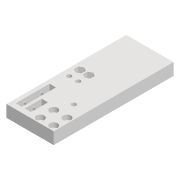
# Autodesk Inventor part: Fixed top coupler
Saved by Autodesk Inventor 2020 (Build 240168000, 168)
## iProperties
Created: 2019-10-02
Part Number: Fixed top coupler
Material: Generic
Document SubType Name: Modeling
Designer: ball
Density: 1 g/cm^3
Appearance: Default
Author: ball
Autodesk Inventor part; units mm, degrees
ref_plane "YZ Plane" through (0, 0, 0) normal (1, 0, 0) x (0, 1, 0)
ref_plane "XZ Plane" through (0, 0, 0) normal (0, 1, 0) x (-1, 0, 0)
ref_plane "XY Plane" through (0, 0, 0) normal (0, 0, 1) x (1, 0, 0)
sketch "Sketch1" plane through (0, 0, 0) normal (0, 1, 0) x (-1, 0, 0)
  line L0 (0, 0) -> (35.5, 0)
  line L1 (35.5, 0) -> (35.5, -90)
  line L2 (35.5, -90) -> (0, -90)
  line L3 (0, -90) -> (0, 0)
  dimension "d0" = 35.5
  dimension "d1" = 90
  constraints: 8 end point, 2 parallel, 1 horizontal, 1 perpendicular
  measures "d0" distance of L1.end L2.end
  measures "d1" distance of L0.end L1.end
extrude "Extrusion1" add sketch "Sketch1" along normal blind 9
sketch "Sketch3" plane through (0, 0, 0) normal (0, -1, 0) x (1, 0, 0)
  circle A0 centre (-10, -25) radius 3.25 construction
  line L0 (0, 0) -> (-35.5, 0) projected
  line L1 (-35.5, 0) -> (-35.5, -90) projected
  line L2 (-11.6286, -27.8125) -> (-13.25, -24.9958)
  line L3 (-13.25, -24.9958) -> (-11.6214, -22.1833)
  line L4 (-11.6214, -22.1833) -> (-8.3714, -22.1875)
  line L5 (-8.3714, -22.1875) -> (-6.75, -25.0042)
  line L6 (-6.75, -25.0042) -> (-8.3786, -27.8167)
  line L7 (-8.3786, -27.8167) -> (-11.6286, -27.8125)
  line L8 (0, -90) -> (0, 0) projected
  dimension "d15" = 6.5
  dimension "d16" = 25
  dimension "d26" = 10
  constraints: 12 end point, 1 coincident, 16 other
  measures "d16" distance from line of L0 point (-10, -25)
  measures "d26" distance from line of L8 point (-10, -25)
extrude "Extrusion3" cut sketch "Sketch3" against normal blind 5
sketch "Sketch5" plane through (0, 9, 0) normal (0, 1, 0) x (1, 0, 0)
  line L0 (0, 0) -> (0, 90) projected
  line L1 (-35.5, 0) -> (0, 0) projected
  circle A0 centre (-10, 25) radius 1.7
  dimension "d36" = 3.4
  dimension "d37" = 25
  constraints: 1 centre point
  measures "d36" diameter of A0
  measures "d37" distance from line of L1 A0.centre
extrude "Extrusion4" cut sketch "Sketch5" against normal through all
sketch "Sketch6" plane through (0, 9, 0) normal (0, 1, 0) x (1, 0, 0)
  line L0 (-32.5, 4) -> (-27.7502, 4)
  line L1 (-27.7502, 4) -> (-27.7502, 29.4)
  line L2 (-27.7502, 29.4) -> (-32.5, 29.4)
  line L3 (-32.5, 29.4) -> (-32.5, 4)
  line L4 (-35.5, 0) -> (0, 0) projected
  line L5 (-35.5, 90) -> (-35.5, 0) projected
  line L6 (-25.7502, 4) -> (-21.0002, 4)
  line L7 (-21.0002, 4) -> (-21.0002, 16.7)
  line L8 (-21.0002, 16.7) -> (-25.7502, 16.7)
  line L9 (-25.7502, 16.7) -> (-25.7502, 4)
  line L10 (0, 0) -> (0, 90) construction
  line L11 (-35.5, 90) -> (0, 90) projected
  line L12 (0, 0) -> (-20, 0) construction
  line L13 (-20, 0) -> (-20, 90) construction
  line L14 (-20, 90) -> (0, 90) construction
  line L15 (0, 90) -> (0, 0)
  circle A0 centre (-23.3752, 41.7) radius 1.7
  circle A1 centre (-30.125, 41.7) radius 1.7
  circle A2 centre (-30.125, 49.7) radius 1.7
  circle A3 centre (-23.3752, 49.7) radius 1.7
  dimension "d43" = 4.7498
  dimension "d44" = 25.4
  dimension "d45" = 4
  dimension "d46" = 3
  dimension "d47" = 4.75
  dimension "d48" = 2
  dimension "d49" = 20
  dimension "d50" = 3.4
  dimension "d90" = 3.4
  dimension "d91" = 5.375
  dimension "d92" = 3.4
  dimension "d93" = 8
  dimension "d94" = 3.4
  dimension "d99" = 40.3
  constraints: 24 end point, 6 parallel, 4 centre point, 3 horizontal, 3 perpendicular, 1 point on line
  measures "d43" distance of L2.end L1.end
  measures "d44" distance of L1.end L0.end
  measures "d45" distance between parallel lines of L4 L0
  measures "d46" distance between parallel lines of L5 L3
  measures "d47" distance of L8.end L7.end
  measures "d48" distance between parallel lines of L9 L1
  measures "d49" distance of L13.end L14.end
  measures "d50" diameter of A0
  measures "d90" diameter of A1
  measures "d91" distance from line of L5 A1.centre
  measures "d92" diameter of A2
  measures "d93" distance of A2.centre A1.centre
  measures "d94" diameter of A3
  measures "d99" distance from line of L11 A2.centre
extrude "Extrusion5" cut sketch "Sketch6" against normal through all contours L3 L2 L1 L0 | L9 L8 L7 L6 | A0 | A1 | A2 | A3
sketch "Sketch7" plane through (0, 0, 0) normal (0, -1, 0) x (1, 0, 0)
  circle A0 centre (-23.3752, -41.7) radius 1.7 projected
  circle A1 centre (-23.3752, -41.7) radius 3.25 construction
  line L0 (-23.3752, -38.45) -> (-20.5606, -40.075)
  line L1 (-20.5606, -40.075) -> (-20.5606, -43.325)
  line L2 (-20.5606, -43.325) -> (-23.3752, -44.95)
  line L3 (-23.3752, -44.95) -> (-26.1898, -43.325)
  line L4 (-26.1898, -43.325) -> (-26.1898, -40.075)
  line L5 (-26.1898, -40.075) -> (-23.3752, -38.45)
  line L6 (0, 0) -> (-35.5, 0) projected
  circle A2 centre (-30.125, -41.7) radius 3.25 construction
  line L7 (-35.5, 0) -> (-35.5, -90) projected
  line L8 (-30.1645, -44.9498) -> (-32.9591, -43.2907)
  line L9 (-32.9591, -43.2907) -> (-32.9196, -40.0409)
  line L10 (-32.9196, -40.0409) -> (-30.0855, -38.4502)
  line L11 (-30.0855, -38.4502) -> (-27.2909, -40.1093)
  line L12 (-27.2909, -40.1093) -> (-27.3304, -43.3591)
  line L13 (-27.3304, -43.3591) -> (-30.1645, -44.9498)
  dimension "d88" = 6.5
  dimension "d54" = 6.5
  dimension "d87" = 41.7
  dimension "d89" = 5.375
  constraints: 24 end point, 3 coincident, 1 centre point, 17 other
  measures "d54" diameter of A1
  measures "d87" distance from line of L6 A1.centre
  measures "d89" distance from line of L7 point (-30.125, -41.7)
extrude "Extrusion6" cut sketch "Sketch7" against normal blind 5
sketch "Sketch8" plane through (-35.5, 0, -90) normal (-1, 0, 0) x (0, 0, 1)
  circle A0 centre (79.65, 4.5) radius 1.4605
  line L0 (0, 9) -> (90, 9) projected
  line L1 (90, 0) -> (90, 9) projected
  circle A1 centre (66.95, 4.5) radius 1.4605
  dimension "d57" = 2.921
  dimension "d58" = 4.5
  dimension "d59" = 10.35
  dimension "d103" = 2.921
  dimension "d104" = 4.5
  dimension "d105" = 12.7
  constraints: 2 centre point
  measures "d57" diameter of A0
  measures "d58" distance from line of L0 A0.centre
  measures "d59" distance from line of L1 A0.centre
  measures "d103" diameter of A1
  measures "d104" distance from line of L0 A1.centre
  measures "d105" distance of A0.centre A1.centre
hole "Hole1" at (-35.5, 4.5, -10.35) at (-35.5, 4.5, -23.05) direction (1, 0, 0) diameter 2.921 depth 21 counterbore diameter 3.4 counterbore depth 1.5
sketch "Sketch9" plane through (-21.0002, 9, -16.7) normal (-1, 0, 0) x (0, 0, 1)
  circle A0 centre (6.35, -4.5) radius 1.4605 projected
  circle A1 centre (6.35, -4.5) radius 2.54
  point P0 (16.7, -9)
  dimension "d67" = 5.08
  constraints: 1 centre point, 1 coincident
  measures "d67" diameter of A1
extrude "Extrusion7" add sketch "Sketch9" along normal blind 0.2032
sketch "Sketch10" plane through (-27.7502, 9, -29.4) normal (-1, 0, 0) x (0, 0, 1)
  circle A0 centre (6.35, -4.5) radius 1.7 projected
  circle A1 centre (6.35, -4.5) radius 2.54
  circle A2 centre (19.05, -4.5) radius 2.54 projected
  circle A3 centre (19.05, -4.5) radius 2.54
  circle A4 centre (19.05, -4.5) radius 1.7
  point P0 (29.4, -9)
  dimension "d70" = 5.08
  dimension "d106" = 3.4
  constraints: 3 centre point, 3 coincident
  measures "d70" diameter of A1
  measures "d106" diameter of A4
extrude "Extrusion8" add sketch "Sketch10" along normal blind 0.2032
sketch "Sketch11" plane through (-25.7502, 9, -4) normal (1, 0, 0) x (0, 0, -1)
  circle A0 centre (6.35, -4.5) radius 1.7 projected
  circle A1 centre (6.35, -4.5) radius 2.54
  point P0 (-4, -9)
  dimension "d73" = 5.08
  constraints: 1 centre point, 1 coincident
  measures "d73" diameter of A1
extrude "Extrusion9" add sketch "Sketch11" along normal blind 0.2032
sketch "Sketch12" plane through (-32.5, 9, -4) normal (1, 0, 0) x (0, 0, -1)
  circle A0 centre (6.35, -4.5) radius 1.7 projected
  circle A1 centre (6.35, -4.5) radius 2.54
  circle A2 centre (19.05, -4.5) radius 1.4605 projected
  circle A3 centre (19.05, -4.5) radius 2.54
  circle A4 centre (19.05, -4.5) radius 1.7
  point P0 (-4, -9)
  dimension "d76" = 5.08
  dimension "d107" = 5.08
  dimension "d108" = 3.4
  constraints: 3 centre point, 3 coincident
  measures "d76" diameter of A1
  measures "d107" diameter of A3
  measures "d108" diameter of A4
extrude "Extrusion10" add sketch "Sketch12" along normal blind 0.2032 contours A1 | A3
sketch "Sketch14" plane through (0, 0, -90) normal (0, 0, -1) x (-1, 0, 0)
  circle A0 centre (18, 4.5) radius 2.25
  line L0 (35.5, 0) -> (0, 0) projected
  line L1 (0, 0) -> (0, 9) projected
  dimension "d82" = 4.5
  dimension "d83" = 4.5
  dimension "d84" = 18
  constraints: 1 centre point
  measures "d82" diameter of A0
  measures "d83" distance from line of L0 A0.centre
  measures "d84" distance from line of L1 A0.centre
extrude "Extrusion11" cut sketch "Sketch14" against normal blind 41
sketch "Sketch15" plane through (0, 9, 0) normal (0, 1, 0) x (1, 0, 0)
  circle A0 centre (-30.125, 49.7) radius 1.7 projected
  circle A1 centre (-30.125, 49.7) radius 3.25 construction
  circle A2 centre (-23.3752, 49.7) radius 1.7 projected
  circle A3 centre (-23.3752, 49.7) radius 3.25 construction
  line L0 (-30.125, 52.95) -> (-27.3104, 51.325)
  line L1 (-27.3104, 51.325) -> (-27.3104, 48.075)
  line L2 (-27.3104, 48.075) -> (-30.125, 46.45)
  line L3 (-30.125, 46.45) -> (-32.9396, 48.075)
  line L4 (-32.9396, 48.075) -> (-32.9396, 51.325)
  line L5 (-32.9396, 51.325) -> (-30.125, 52.95)
  line L6 (-23.3752, 52.95) -> (-20.5606, 51.325)
  line L7 (-20.5606, 51.325) -> (-20.5606, 48.075)
  line L8 (-20.5606, 48.075) -> (-23.3752, 46.45)
  line L9 (-23.3752, 46.45) -> (-26.1898, 48.075)
  line L10 (-26.1898, 48.075) -> (-26.1898, 51.325)
  line L11 (-26.1898, 51.325) -> (-23.3752, 52.95)
  point P0 (0, 0)
  dimension "d95" = 6.5
  dimension "d96" = 6.5
  constraints: 24 end point, 4 coincident, 2 vertical alignment, 30 other
extrude "Extrusion12" cut sketch "Sketch15" against normal blind 5
sketch "Sketch17" plane through (0, 9, 0) normal (0, 1, 0) x (1, 0, 0)
  arc A0 (-2.6064, 3.3135) -> (-3.3135, 2.6064) centre (-3.77, 3.77) ccw construction
  arc A1 (-14.2265, 2.6064) -> (-14.9336, 3.3135) centre (-13.77, 3.77) ccw construction
  arc A2 (-14.9336, 14.2265) -> (-14.2265, 14.9336) centre (-13.77, 13.77) ccw construction
  arc A3 (-3.3135, 14.9336) -> (-2.6064, 14.2265) centre (-3.77, 13.77) ccw construction
  point P0 (0, 0)
hole "Hole2" at (-3.77, 9, -3.77) at (-13.77, 9, -3.77) at (-13.77, 9, -13.77) at (-3.77, 9, -13.77) direction (0, -1, 0) diameter 3.4 end through all counterbore diameter 5.9 counterbore depth 3.5
body "Solid1"
